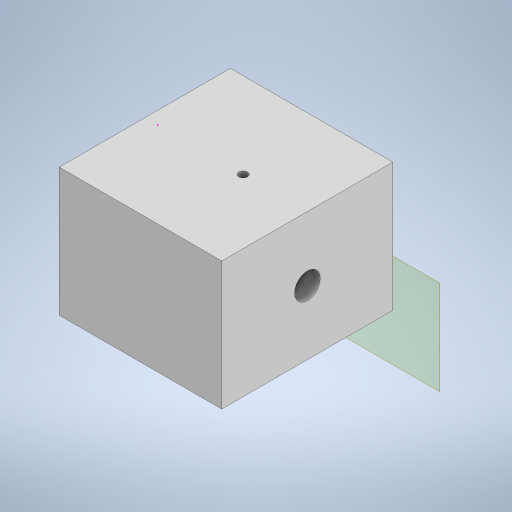
# Autodesk Inventor part: magnet_test_print
Saved by Autodesk Inventor 2023 (Build 270158000, 158)
## iProperties
Created: 2021-04-13
Part Number: magnet_test_print
Material: Generic
Document SubType Name: Modeling
Designer: KAMPFF-LAB-BEHAVIOR
Density: 1 g/cm^3
Appearance: Default
Author: KAMPFF-LAB-BEHAVIOR
Autodesk Inventor part; units mm, degrees
ref_plane "YZ Plane" through (0, 0, 0) normal (1, 0, 0) x (0, 1, 0)
ref_plane "XZ Plane" through (0, 0, 0) normal (0, 1, 0) x (-1, 0, 0)
ref_plane "XY Plane" through (0, 0, 0) normal (0, 0, 1) x (1, 0, 0)
ref_plane "Work Plane13" through (0, 3, 0) normal (0, 1, 0) x (1, 0, 0)
sketch "Sketch45" plane through (0, 3, 0) normal (0, 1, 0) x (1, 0, 0)
  line L0 (35, -20) -> (-3, -20)
  line L1 (-3, -20) -> (-3, 20)
  line L2 (-3, 20) -> (35, 20)
  line L3 (35, 20) -> (35, -20)
  point P0 (0, 0)
  dimension "d142" = 38
  dimension "d143" = 40
  constraints: 8 end point, 2 parallel, 1 horizontal, 1 perpendicular
  measures "d142" distance of L1.end L2.end
  measures "d143" distance of L0.end L1.end
extrude "Extrusion34" add sketch "Sketch45" along normal blind 30
sketch "Sketch46" plane through (0, 33, 0) normal (0, 1, 0) x (1, 0, 0)
  point P0 (0, 0)
ref_plane "Work Plane11" through (0, 0, 0) normal (0, -1, 0) x (1, 0, 0)
sketch "Sketch47" plane through (0, 0, 0) normal (0, -1, 0) x (1, 0, 0)
  circle A0 centre (16, 0) radius 18
  point P0 (0, 0)
  dimension "d146" = 36
  constraints: 1 centre point
  measures "d146" diameter of A0
extrude "Extrusion35" cut sketch "Sketch47" against normal blind 30 draft -15
sketch "Sketch48" plane through (0, 33, 0) normal (0, 1, 0) x (1, 0, 0)
  point P0 (0, 0)
sketch "Sketch49" plane through (0, 33, 0) normal (0, 1, 0) x (1, 0, 0)
  circle A0 centre (20, 0) radius 1
  point P0 (0, 0)
  dimension "d149" = 2
  constraints: 1 centre point
  measures "d149" diameter of A0
extrude "Extrusion36" cut sketch "Sketch49" against normal through all
ref_plane "Work Plane7" through (35, 3, -20) normal (0, 0, -1) x (-1, 0, 0)
sketch "Sketch58" plane through (35, 3, -20) normal (0, 0, -1) x (-1, 0, 0)
  line L0 (7, 20) -> (27, 20)
  line L1 (27, 20) -> (27, 5)
  line L2 (27, 5) -> (7, 5)
  line L3 (7, 5) -> (7, 20)
  point P0 (35, -3)
  dimension "d156" = 20
  dimension "d157" = 15
  constraints: 8 end point, 2 parallel, 1 horizontal, 1 perpendicular
  measures "d156" distance of L1.end L2.end
  measures "d157" distance of L0.end L1.end
extrude "Extrusion38" cut sketch "Sketch58" against normal blind 15
ref_plane "Work Plane4" through (-3, 3, -20) normal (-1, 0, 0) x (0, 0, 1)
sketch "Sketch59" plane through (-3, 3, -20) normal (-1, 0, 0) x (0, 0, 1)
  line L0 (4.8, 25) -> (8, 25)
  line L1 (8, 25) -> (8, 5)
  line L2 (8, 5) -> (4.8, 5)
  line L3 (4.8, 5) -> (4.8, 25)
  point P0 (20, -3)
  dimension "d160" = 3.2
  dimension "d161" = 20
  constraints: 8 end point, 2 parallel, 1 horizontal, 1 perpendicular
  measures "d160" distance of L1.end L2.end
  measures "d161" distance of L0.end L1.end
extrude "Extrusion39" cut sketch "Sketch59" against normal blind 35
ref_plane "Work Plane1" through (0, 3, 0) normal (0, 1, 0) x (1, 0, 0)
ref_plane "Work Plane6" through (0, 23, 0) normal (0, 1, 0) x (1, 0, 0)
sketch "Sketch62" plane through (-3, 3, -20) normal (-1, 0, 0) x (0, 0, 1)
  circle A0 centre (20, 15) radius 3
  point P0 (20, -3)
  dimension "d172" = 6
  constraints: 1 centre point
  measures "d172" diameter of A0
extrude "Extrusion42" cut sketch "Sketch62" against normal through all
sketch "Sketch65" plane through (0, 3, 0) normal (0, -1, 0) x (1, 0, 0)
  line L0 (-3, -12) -> (32, -12) projected
  line L1 (28, -20) -> (28, -15.2) projected
  line L2 (3.5815, -12) -> (28, -12)
  line L3 (28, -12) -> (28, -17.2375)
  line L4 (28, -17.2375) -> (3.5815, -17.2375)
  line L5 (3.5815, -17.2375) -> (3.5815, -12)
  point P0 (0, 0)
  constraints: 8 end point, 2 parallel, 2 point on line, 1 horizontal, 1 perpendicular
extrude "Extrusion44" add sketch "Sketch65" against normal blind 5
body "Solid9"
